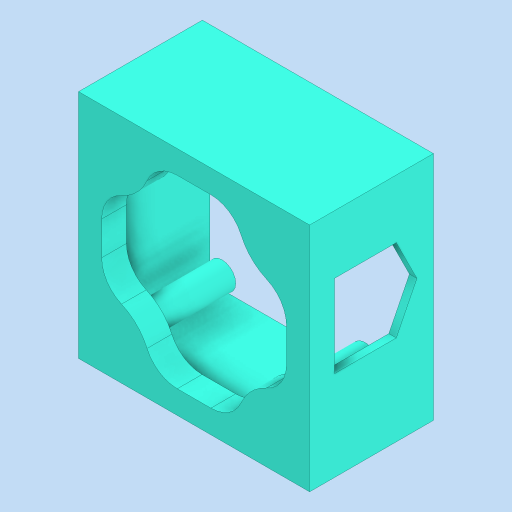
# Autodesk Inventor part: BackSide
Saved by Autodesk Inventor 2024 (Build 280153000, 153)
## iProperties
Created: 2020-01-17
Part Number: BackSide
Material: Generic
Document SubType Name: Modeling
Designer: Conrad
Density: 1 g/cm^3
Appearance: Default
Author: Conrad
## iProperties of the stored document V2_MountHousing_3DPrint.ipt
Created: 2024-02-20
Part Number: V2_MountHousing_3DPrint
Material: Generic
Document SubType Name: Modeling
Designer: mones
Density: 1 g/cm^3
Appearance: Default
Author: mones
Autodesk Inventor part; units mm, degrees
ref_plane "YZ Plane" through (0, 0, 0) normal (1, 0, 0) x (0, 1, 0)
ref_plane "XZ Plane" through (0, 0, 0) normal (0, 1, 0) x (-1, 0, 0)
sketch "Sketch1" plane through (0, 0, 0) normal (0, 0, 1) x (1, 0, 0)
  line L0 (33.1238, 20.8366) -> (-2.4362, 20.8366)
  line L1 (-2.4362, 20.8366) -> (-2.4362, -14.7234)
  line L2 (-2.4362, -14.7234) -> (33.1238, -14.7234)
  line L3 (33.1238, -14.7234) -> (33.1238, 20.8366)
  circle A0 centre (4.3476, -7.9396) radius 1.0922
  circle A1 centre (26.34, -7.9396) radius 1.0922
  circle A2 centre (4.3476, 14.0528) radius 1.0922
  circle A3 centre (26.34, 14.0528) radius 1.0922
  line L4 (32.4234, 14.0528) -> (-3.1366, 14.0528) construction
  line L5 (31.7464, -7.9396) -> (-3.8136, -7.9396) construction
  line L6 (4.3476, 22.271) -> (4.3476, -13.289) construction
  line L7 (26.34, 20.1424) -> (26.34, -15.4176) construction
  point P0 (0, 0)
  dimension "CameraHole" = 2.1844
  dimension "BaseWidth" = 35.56
  constraints: 16 end point, 8 point on line, 6 parallel, 5 equal length, 4 centre point, 3 equal radius, 1 horizontal, 1 perpendicular, 1 vertical
  measures "CameraHole" diameter of A3
  measures "BaseWidth" distance of L3.start L0.start
extrude "Base" add sketch "Sketch1" along normal blind 3.81
sketch "Sketch2" plane through (0, 0, 0) normal (0, 0, -1) x (-1, 0, 0)
  line L0 (-12.7595, 17.2806) -> (-17.9281, 17.2806)
  line L1 (-29.5678, 5.6408) -> (-29.5678, 0.4723)
  line L2 (-1.1198, 0.4723) -> (-1.1198, 5.6408)
  line L3 (2.4362, 20.8366) -> (2.4362, -14.7234) projected
  line L4 (2.4362, -14.7234) -> (-33.1238, -14.7234) projected
  line L5 (-33.1238, 20.8366) -> (2.4362, 20.8366) projected
  line L6 (-31.3438, -12.9434) -> (-31.3438, 19.0566) construction
  line L7 (-31.3438, 19.0566) -> (0.6562, 19.0566) construction
  line L8 (0.6562, 19.0566) -> (0.6562, -12.9434) construction
  circle A0 centre (-26.34, 14.0528) radius 1.0922 construction
  line L9 (-1.041, 19.0566) -> (-1.041, 20.8366) construction
  line L10 (-1.1198, 17.2806) -> (-29.5678, 17.2806)
  line L11 (-29.5678, 17.2806) -> (-29.5678, -11.1674)
  line L12 (-17.9281, -11.1674) -> (-12.7595, -11.1674)
  line L13 (-1.1198, -11.1674) -> (-1.1198, 17.2806)
  arc A1 (-26.5198, 10.2967) -> (-22.584, 14.2326) centre (-29.5678, 17.2806) ccw
  arc A2 (-22.584, -8.1194) -> (-26.5198, -4.1836) centre (-29.5678, -11.1674) ccw
  arc A3 (-4.1678, -4.1836) -> (-8.1037, -8.1194) centre (-1.1198, -11.1674) ccw
  arc A4 (-8.1037, 14.2326) -> (-4.1678, 10.2967) centre (-1.1198, 17.2806) ccw
  arc A5 (-29.5678, 0.4723) -> (-26.5198, -4.1836) centre (-24.4878, 0.4723) ccw
  arc A6 (-26.5198, 10.2967) -> (-29.5678, 5.6408) centre (-24.4878, 5.6408) ccw
  arc A7 (-17.9281, 17.2806) -> (-22.584, 14.2326) centre (-17.9281, 12.2006) ccw
  arc A8 (-8.1037, 14.2326) -> (-12.7595, 17.2806) centre (-12.7595, 12.2006) ccw
  arc A9 (-1.1198, 5.6408) -> (-4.1678, 10.2967) centre (-6.1998, 5.6408) ccw
  arc A10 (-4.1678, -4.1836) -> (-1.1198, 0.4723) centre (-6.1998, 0.4723) ccw
  arc A11 (-12.7595, -11.1674) -> (-8.1037, -8.1194) centre (-12.7595, -6.0874) ccw
  arc A12 (-22.584, -8.1194) -> (-17.9281, -11.1674) centre (-17.9281, -6.0874) ccw
  point P0 (-29.5678, 9.6606)
  point P1 (-21.9478, 17.2806)
  point P2 (-21.9478, -11.1674)
  point P3 (-29.5678, -3.5474)
  point P4 (-1.1198, -3.5474)
  point P5 (-8.7398, -11.1674)
  point P6 (-8.7398, 17.2806)
  point P7 (-1.1198, 9.6606)
  dimension "d13" = 3.556
  dimension "d16" = 3.556
  dimension "d38" = 32
  dimension "d101" = 28.448
  dimension "d102" = 7.62
  dimension "d103" = 7.62
  dimension "d104" = 7.62
  dimension "d105" = 7.62
  dimension "d106" = 5.08
  constraints: 32 point on circle, 22 end point, 16 point on line, 16 tangent, 12 centre point, 7 equal radius, 4 coincident, 4 parallel, 4 perpendicular, 1 collinear, 1 horizontal
  measures "d13" distance between parallel lines of L3 L2
  measures "d16" distance between parallel lines of L5 L0
  measures "d38" distance of L6.end L7.end
  measures "d101" distance of L11.end L10.end
  measures "d102" radius of A1
  measures "d103" radius of A2
  measures "d104" radius of A3
  measures "d105" radius of A4
  measures "d106" radius of A5
extrude "Open Back" cut sketch "Sketch2" against normal blind 3.81 contours A8 A4 A9 L2 A10 A3 A11 L12 A12 A2 A5 L1 A6 A1 A7 L0
sketch "Sketch4" plane through (0, 0, 0) normal (0, 0, -1) x (-1, 0, 0)
  line L0 (-33.1238, 20.8366) -> (2.4362, 20.8366)
  line L1 (2.4362, 20.8366) -> (2.4362, -14.7234)
  line L2 (2.4362, -14.7234) -> (-33.1238, -14.7234)
  line L3 (-33.1238, -14.7234) -> (-33.1238, 20.8366)
  line L4 (1.2932, -13.5804) -> (-31.9808, -13.5804)
  line L5 (-31.9808, -13.5804) -> (-31.9808, 19.6936)
  line L6 (-31.9808, 19.6936) -> (1.2932, 19.6936)
  line L7 (1.2932, 19.6936) -> (1.2932, -13.5804)
  point P0 (0, 0)
  dimension "d32" = 1.143
  dimension "d33" = 1.143
  dimension "d34" = 1.143
  dimension "d35" = 1.143
  constraints: 16 end point, 4 parallel, 2 horizontal, 2 perpendicular
  measures "d32" distance between parallel lines of L0 L6
  measures "d33" distance between parallel lines of L1 L7
  measures "d34" distance between parallel lines of L4 L2
  measures "d35" distance between parallel lines of L5 L3
extrude "Housing" add sketch "Sketch4" along normal blind 15.24
ref_plane "Work Plane1" through (0, 0, -15.24) normal (0, 0, -1) x (-1, 0, 0)
sketch "Sketch10" plane through (0, 0, 3.81) normal (0, 0, 1) x (1, 0, 0)
  circle A0 centre (4.3476, 14.0528) radius 1.0922 projected
  circle A1 centre (4.3476, 14.0528) radius 1.0922
  circle A2 centre (4.3476, -7.9396) radius 1.0922 projected
  circle A3 centre (4.3476, -7.9396) radius 1.0922
  circle A4 centre (26.34, -7.9396) radius 1.0922 projected
  circle A5 centre (26.34, -7.9396) radius 1.0922
  circle A6 centre (26.34, 14.0528) radius 1.0922 projected
  circle A7 centre (26.34, 14.0528) radius 1.0922
  point P0 (0, 0)
  constraints: 4 centre point, 4 coincident
extrude "HoleClosing" add sketch "Sketch10" against normal blind 1.27
sketch "Sketch15" plane through (33.1238, -14.7234, 3.81) normal (1, 0, 0) x (0, 0, -1)
  line L0 (3.81, 34.417) -> (19.05, 34.417) projected
  line L1 (3.81, 34.417) -> (3.81, 1.143) projected
  line L2 (3.81, 1.143) -> (19.05, 1.143) projected
  line L3 (19.05, 34.417) -> (19.05, 1.143) projected
  line L4 (19.05, 34.417) -> (10.16, 34.417)
  line L5 (10.16, 34.417) -> (10.16, 20.193)
  line L6 (13.335, 13.843) -> (3.81, 13.843)
  line L7 (3.81, 13.843) -> (3.81, 26.543)
  line L8 (3.81, 26.543) -> (13.335, 26.543)
  line L9 (10.16, 26.543) -> (13.335, 26.543)
  line L10 (13.335, 26.543) -> (16.51, 20.193)
  line L11 (16.51, 20.193) -> (13.335, 13.843)
  line L12 (10.16, 20.193) -> (3.81, 26.543) construction
  line L13 (10.16, 20.193) -> (3.81, 13.843) construction
  point P0 (3.81, 26.543)
  point P1 (3.81, 13.843)
  dimension "d107" = 8.89
  dimension "d108" = 14.224
  constraints: 20 end point, 2 point on line, 1 collinear, 1 parallel, 1 perpendicular
  measures "d107" distance of L0.end L4.end
  measures "d108" distance of L5.end L4.end
extrude "Cable Hole" cut sketch "Sketch15" against normal blind 3.81 contours L8 L10 L11 L6 L1
sketch "Sketch3" plane through (0, 0, 0) normal (0, 0, -1) x (-1, 0, 0)
  circle A0 centre (-4.3476, -7.9396) radius 1.143
  circle A1 centre (-4.3476, -7.9396) radius 2.0805
  circle A2 centre (-4.3476, -7.9396) radius 1.0922 projected
  line L0 (-19.1558, -6.3775) -> (-19.1558, -11.4067) projected
  circle A3 centre (-4.3476, 14.0528) radius 1.143
  circle A4 centre (-4.3476, 14.0528) radius 2.0828
  circle A5 centre (-4.3476, 14.0528) radius 1.0922 projected
  circle A6 centre (-26.34, 14.0528) radius 2.0828
  circle A7 centre (-26.34, 14.0528) radius 1.143
  circle A8 centre (-26.34, 14.0528) radius 1.0922 projected
  arc A9 (-24.3548, -7.3094) -> (-25.3959, -9.7962) centre (-26.34, -7.9396) ccw
  circle A10 centre (-26.34, -7.9396) radius 1.143
  circle A11 centre (-26.34, -7.9396) radius 1.0922 projected
  circle A12 centre (-26.34, -7.9396) radius 2.0828
  point P0 (0, 0)
  point P1 (-24.3548, -7.3094)
  dimension "d21" = 0.9375
  dimension "d26" = 2.286
  dimension "d30" = 2.286
  dimension "d31" = 0.9398
  constraints: 8 centre point, 5 coincident, 4 concentric, 4 equal radius, 2 point on circle, 3 other
  measures "d21" radial gap between concentric circles of A1 A0
  measures "d26" diameter of A0
  measures "d30" diameter of A3
  measures "d31" radial gap between concentric circles of A3 A4
extrude "Pegs" add sketch "Sketch3" along normal blind 11.5062 contours A1 | A4 | A6 | A12 A9
sketch "Sketch16" plane through (31.9808, -13.5804, -15.24) normal (-1, 0, 0) x (0, 0, 1)
  line L0 (15.24, 3.558) -> (3.7338, 3.558) projected
  line L1 (15.24, 7.7236) -> (3.7338, 7.7236) projected
  line L2 (3.7338, 7.7236) -> (3.7338, 3.558)
  line L3 (15.24, 12.7) -> (15.24, 0) projected
  line L4 (3.7338, 7.7236) -> (15.24, 7.7236)
  line L5 (15.24, 7.7236) -> (15.24, 3.558)
  line L6 (15.24, 3.558) -> (3.7338, 3.558)
  circle A0 centre (10.4775, 5.6408) radius 2.0828
  line L7 (12.065, 10.414) -> (12.065, 6.9891)
  line L8 (12.065, 4.2925) -> (12.065, 0)
  line L9 (15.24, 5.6408) -> (12.5603, 5.6408)
  line L10 (8.3947, 5.6408) -> (3.7338, 5.6408)
  line L11 (10.4775, 10.414) -> (10.4775, 7.7236)
  line L12 (10.4775, 3.558) -> (10.4775, 0)
  line L13 (8.89, 10.414) -> (8.89, 6.9891)
  line L14 (8.89, 4.2925) -> (8.89, 0)
  line L15 (10.4775, 5.6408) -> (10.4775, 27.6372)
  circle A1 centre (10.4775, 27.6372) radius 2.0828
  dimension "d116" = 21.9964
  dimension "d117" = 4.1656
  constraints: 26 end point, 12 parallel, 2 perpendicular, 1 centre point, 1 coincident, 1 collinear, 1 horizontal, 1 point on line, 1 vertical, 10 other
  measures "d116" distance of L15.start L15.end
  measures "d117" diameter of A1
extrude "Zip-Tie Attachment" add sketch "Sketch16" along normal blind 5.6388 contours A1
sketch "Sketch17" plane through (26.34, 14.0528, -11.5062) normal (0, 0, -1) x (-1, 0, 0)
  circle A0 centre (0, 0) radius 1.143 projected
  circle A1 centre (0, 0) radius 1.143
  constraints: 1 centre point, 1 coincident, 1 concentric
extrude "top left hole" cut sketch "Sketch17" against normal blind 11.5062
equation "\"CameraHole\" = CameraHole_1"
equation "\"BaseWidth\" = BaseWidth_1"
equation "\"d16\" = UsbHoletoWall"
equation "\"BaseWidth_1\" = 35.56"
equation "\"CameraHole_1\" = 2.1844"
equation "\"ZiptieHole\" = 5.08"
equation "\"ZiptieHoletoHoleDistance\" = 2 * ZiptieRadius + WireThickness"
equation "\"WireThickness\" = 4.064"
equation "\"ZiptieRadius\" = 2.54"
equation "\"ZiptieToSide\" = 8.89"
equation "\"UsbHoletoWall\" = 3.556"
equation "\"WasherHolder\" = 12.7"
body "Solid1"
